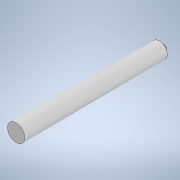
# Autodesk Inventor part: Must
Saved by Autodesk Inventor 2021 (Build 250183000, 183)
## iProperties
Created: 2022-01-12
Part Number: Must
Material: Generic
Document SubType Name: Modeling
Designer: stefi
Density: 1 g/cm^3
Appearance: Default
Author: stefi
Autodesk Inventor part; units mm, degrees
ref_plane "YZ Plane" through (0, 0, 0) normal (1, 0, 0) x (0, 1, 0)
ref_plane "XZ Plane" through (0, 0, 0) normal (0, 1, 0) x (-1, 0, 0)
ref_plane "XY Plane" through (0, 0, 0) normal (0, 0, 1) x (1, 0, 0)
sketch "Sketch1" plane through (0, 0, 0) normal (0, 1, 0) x (-1, 0, 0)
  line L0 (0, 0) -> (0, -340.2)
  line L1 (0, -340.2) -> (7, -340.2)
  line L2 (7, -340.2) -> (7, -330.2)
  line L3 (7, -330.2) -> (18, -330.2)
  line L4 (18, -330.2) -> (20, 0)
  line L5 (20, 0) -> (0, 0)
  dimension "d0" = 10
  dimension "d1" = 18
  dimension "d2" = 7
  dimension "d3" = 330.2
  dimension "d4" = 20
  constraints: 12 end point, 4 perpendicular, 1 vertical
  measures "d0" distance of L1.end L2.end
  measures "d1" horizontal distance of L0.end L3.end
  measures "d2" distance of L1.end L0.end
  measures "d3" vertical distance of L4.end L3.end
  measures "d4" distance of L0.start L4.end
revolve "Revolution1" add sketch "Sketch1" angle 360 about axis through (0, 0, 0) along (0, 0, -1)
chamfer "Chamfer1" distance 0.5 angle 45 1 edges at (7, 0, -340.2)
body "Solid1"
